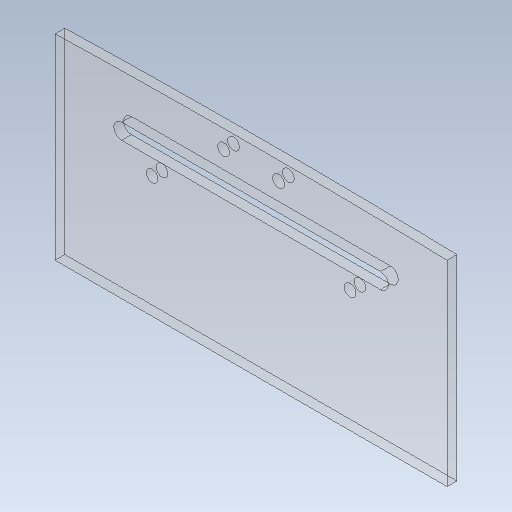
# Autodesk Inventor part: platform_part
Saved by Autodesk Inventor 2020 (Build 240168000, 168)
## iProperties
Created: 2019-10-02
Part Number: platform_part
Material: Generic
Document SubType Name: Modeling
Designer: ZEUSLAP
Density: 1 g/cm^3
Appearance: Default
Author: ZEUSLAP
Autodesk Inventor part; units mm, degrees
ref_plane "YZ Plane" through (0, 0, 0) normal (1, 0, 0) x (0, 1, 0)
ref_plane "XZ Plane" through (0, 0, 0) normal (0, 1, 0) x (-1, 0, 0)
ref_plane "XY Plane" through (0, 0, 0) normal (0, 0, 1) x (1, 0, 0)
sketch "Sketch1" plane through (0, 0, 0) normal (0, 0, 1) x (1, 0, 0)
  line L0 (-50, 25) -> (50, 25)
  line L1 (50, 25) -> (50, -25)
  line L2 (50, -25) -> (-50, -25)
  line L3 (-50, -25) -> (-50, 25)
  line L4 (-35, 12) -> (35, 12) construction
  line L5 (-33, 10) -> (33, 10)
  line L6 (33, 14) -> (-33, 14)
  arc A0 (-33, 14) -> (-33, 10) centre (-33, 12) ccw
  arc A1 (33, 10) -> (33, 14) centre (33, 12) ccw
  arc A2 (50, 25) -> (-50, 25) centre (0, -1974.3749) ccw
  circle A3 centre (-25.25, 6) radius 1.5
  circle A4 centre (25.25, 6) radius 1.5
  circle A5 centre (-7, 21) radius 1.5
  circle A6 centre (7, 21) radius 1.5
  line L7 (0, 134.945) -> (0, -92.5364) construction
  point P0 (0, 0)
  point P1 (50, 0)
  point P2 (0, -25)
  point P3 (0, 12)
  point P4 (35, 25.3188)
  point P5 (35, 6)
  dimension "d0" = 50
  dimension "d1" = 100
  dimension "d2" = 4
  dimension "d4" = 66
  dimension "d5" = 2000
  dimension "d6" = 50.5
  dimension "d7" = 3
  dimension "d8" = 14
  dimension "d9" = 9
  dimension "d10" = 4
  dimension "d11" = 6
  dimension "d14" = 13.3188
  dimension "d15" = 19.3188
  constraints: 18 end point, 10 point on circle, 7 centre point, 4 horizontal alignment, 4 tangent, 4 vertical alignment, 3 equal radius, 3 midpoint, 3 parallel, 3 point on line, 2 horizontal, 1 coincident, 1 perpendicular, 1 vertical, 2 other
  measures "d0" distance of L2.end L0.start
  measures "d1" distance of L1.end L2.end
  measures "d2" diameter of A1
  measures "d4" distance of L6.start L6.end
  measures "d5" radius of A2
  measures "d6" distance of A4.centre A3.centre
  measures "d7" diameter of A5
  measures "d8" distance of A6.centre A5.centre
  measures "d9" distance from line of L4 A5.centre
  measures "d10" distance from line of L0 A5.centre
  measures "d11" vertical distance of A3.centre point (0, 12)
  measures "d14" distance of point (35, 12) point (35, 25.319)
  measures "d15" distance of point (35, 25.319) point (35, 6)
extrude "Extrusion1" add sketch "Sketch1" along normal blind 2.5
body "Solid1"
